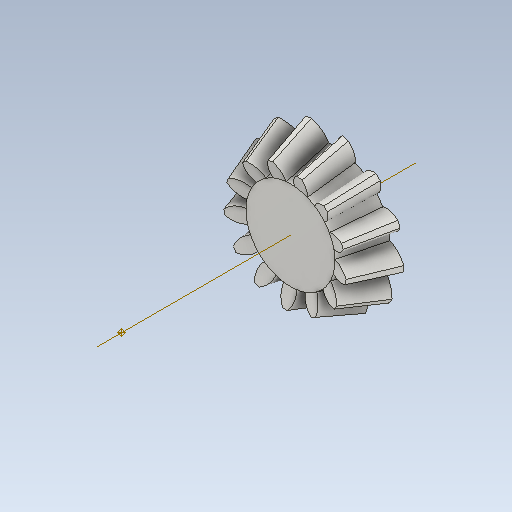
# Autodesk Inventor part: Kegelrad1
Saved by Autodesk Inventor 2021 (Build 250183000, 183)
## iProperties
CustomPartVersion: 1
Created: 2021-01-28
Part Number: Kegelrad1
Material: Steel, Mild
Document SubType Name: Modeling
Designer: LETPJG
Categories: <?xml version="1.0" encoding="UTF-16"?> <MemberInstance><Categories><FamilyTemplate><FamilyTemplateParameter ValueType="xs:double" Id="1" ObjectReferenceKey="da_z" ObjectType="kUserParameterObject"/><FamilyTemplateParameter ValueType="xs:double" Id="2" ObjectReferenceKey="da_b" ObjectType="kUserParameterObject"/><FamilyTemplateParameter ValueType="xs:double" Id="3" ObjectReferenceKey="da_beta" ObjectType="kUserParameterObject"/><FamilyTemplateParameter ValueType="xs:double" Id="4" ObjectReferenceKey="da_dae" ObjectType="kUserParameterObject"/><FamilyTemplateParameter ValueType="xs:double" Id="5" ObjectReferenceKey="da_ve" ObjectType="kUserParameterObject"/><FamilyTemplateParameter ValueType="xs:double" Id="6" ObjectReferenceKey="da_omega" ObjectType="kUserParameterObject"/><FamilyTemplateParameter ValueType="xs:string" Id="7" ObjectReferenceKey="EAIAABAAAAAAHwAAAAAAAIAAAAAAAAAA" ObjectType="83914240" SubObjectId="SurfaceGeometry"/></FamilyTemplate><ParamToTemplateMap><ParamToTemplate CategoryParameter="//CategoryParameter[@InternalName='046C89C9-8512-4d59-83FE-43B91F4F132A']" TemplateParameter="1"/><ParamToTemplate CategoryParameter="//CategoryParameter[@InternalName='2552DF32-E462-4b46-AEBF-C6C7768E72AC']" TemplateParameter="2"/><ParamToTemplate CategoryParameter="//CategoryParameter[@InternalName='C9EE641D-15FC-4fae-A226-E94C4372FDD7']" TemplateParameter="3"/><ParamToTemplate><ParamToTemplate CategoryParameter="//CategoryParameter[@InternalName='00B6519A-459B-49c7-AD84-2E56D39A5744']" ConstantValue="0.000000"/></ParamToTemplate><ParamToTemplate><ParamToTemplate CategoryParameter="//CategoryParameter[@InternalName='04B31F0E-C7A6-4894-AA32-9629BEFACF47']" ConstantValue="1.000000"/></ParamToTemplate><ParamToTemplate><ParamToTemplate CategoryParameter="//CategoryParameter[@InternalName='43CBEC2E-7847-49e7-A936-2F7889FCB2D9']" ConstantValue="0.200000"/></ParamToTemplate><ParamToTemplate><ParamToTemplate CategoryParameter="//CategoryParameter[@InternalName='B1EFC894-105D-4ebd-86BF-FA20ED196853']" ConstantValue="0.300000"/></ParamToTemplate><ParamToTemplate><ParamToTemplate CategoryParameter="//CategoryParameter[@InternalName='51175063-3D10-4879-93E8-6246FE8B403D']" ConstantValue="2060000000.000000"/></ParamToTemplate><ParamToTemplate><ParamToTemplate CategoryParameter="//CategoryParameter[@InternalName='A3A52E27-4454-46a9-B0BD-C932399B70AF']" ConstantValue="0.300000"/></ParamToTemplate><ParamToTemplate CategoryParameter="//CategoryParameter[@InternalName='2A200944-5A8C-41ca-B96E-8520D2E510F1']" TemplateParameter="4"/><ParamToTemplate><ParamToTemplate CategoryParameter="//CategoryParameter[@InternalName='1A637F62-92C8-44bc-B81F-10802510B579']" ConstantValue="1.175421"/></ParamToTemplate><ParamToTemplate CategoryParameter="//CategoryParameter[@InternalName='B52DD4BE-6863-48fb-BF58-89EF6F9EC65C']" TemplateParameter="5"/><ParamToTemplate><ParamToTemplate CategoryParameter="//CategoryParameter[@InternalName='3956BFF2-84D2-457d-93C2-9B0613DEBA67']" ConstantValue="1.568105"/></ParamToTemplate><ParamToTemplate CategoryParameter="//CategoryParameter[@InternalName='739CFA02-461B-4bf8-8049-181FCAD8B28F']" TemplateParameter="6"/><ParamToTemplate><ParamToTemplate CategoryParameter="//CategoryParameter[@InternalName='A27E999F-E2CE-4481-8A2A-EBF499C4C3C5']" ConstantValue="0.000000"/></ParamToTemplate><ParamToTemplate><ParamToTemplate CategoryParameter="//CategoryParameter[@InternalName='9E1B4470-B2D3-4ff1-B813-535BB4CDF51A']" ConstantValue="3520000.000000"/></ParamToTemplate><ParamToTemplate><ParamToTemplate CategoryParameter="//CategoryParameter[@InternalName='F8452263-BFF6-458c-9FB1-07C4B99E95CD']" ConstantValue="11400000.000000"/></ParamToTemplate><ParamToTemplate><ParamToTemplate CategoryParameter="//CategoryParameter[@InternalName='3E3BB259-FD49-497f-8171-6EBC954A3479']" ConstantValue="2.000000"/></ParamToTemplate><ParamToTemplate CategoryParameter="//CategoryParameter[@InternalName='27C3BAF2-7550-4e4b-AE2C-0DB134B7D9B7']" TemplateParameter="7"/></ParamToTemplateMap><Category DisplayName="Gear" InternalName="DC85795E-93AB-48d5-8EEE-5A27447B64BD" Mnemonic="Gear"><CategoryParameter DisplayName="z" InternalName="046C89C9-8512-4d59-83FE-43B91F4F132A" Mnemonic="z"/><CategoryParameter DisplayName="b" InternalName="2552DF32-E462-4b46-AEBF-C6C7768E72AC" Mnemonic="b"/><CategoryParameter DisplayName="||b|" InternalName="C9EE641D-15FC-4fae-A226-E94C4372FDD7" Mnemonic="beta"/><CategoryParameter DisplayName="x" InternalName="00B6519A-459B-49c7-AD84-2E56D39A5744" Mnemonic="x"/><CategoryParameter DisplayName="a*" InternalName="04B31F0E-C7A6-4894-AA32-9629BEFACF47" Mnemonic="a"/><CategoryParameter DisplayName="c*" InternalName="43CBEC2E-7847-49e7-A936-2F7889FCB2D9" Mnemonic="c"/><CategoryParameter DisplayName="r|.f|*" InternalName="B1EFC894-105D-4ebd-86BF-FA20ED196853" Mnemonic="rf"/><CategoryParameter DisplayName="E" InternalName="51175063-3D10-4879-93E8-6246FE8B403D" Mnemonic="E"/><CategoryParameter DisplayName="||m|" InternalName="A3A52E27-4454-46a9-B0BD-C932399B70AF" Mnemonic="mi"/><Category DisplayName="BevelGear" InternalName="0C98F69A-0C2B-4791-B2FE-7691BB227E77" Mnemonic="BevelGear"><CategoryParameter DisplayName="d|.ae|" InternalName="2A200944-5A8C-41ca-B96E-8520D2E510F1" Mnemonic="dae"/><CategoryParameter DisplayName="d|.ai|" InternalName="1A637F62-92C8-44bc-B81F-10802510B579" Mnemonic="dai"/><CategoryParameter DisplayName="A|.e|" InternalName="B52DD4BE-6863-48fb-BF58-89EF6F9EC65C" Mnemonic="ve"/><CategoryParameter DisplayName="A|.i|" InternalName="3956BFF2-84D2-457d-93C2-9B0613DEBA67" Mnemonic="vi"/><CategoryParameter DisplayName="||S|" InternalName="739CFA02-461B-4bf8-8049-181FCAD8B28F" Mnemonic="omega"/><CategoryParameter DisplayName="x|.t|" InternalName="A27E999F-E2CE-4481-8A2A-EBF499C4C3C5" Mnemonic="xt"/><CategoryParameter DisplayName="||s||.Flim|" InternalName="9E1B4470-B2D3-4ff1-B813-535BB4CDF51A" Mnemonic="sFlim"/><CategoryParameter DisplayName="||s||.Hlim|" InternalName="F8452263-BFF6-458c-9FB1-07C4B99E95CD" Mnemonic="sHlim"/><CategoryParameter DisplayName="Typ" InternalName="3E3BB259-FD49-497f-8171-6EBC954A3479" Mnemonic="type"/><CategoryParameter DisplayName="PitchDiameter" InternalName="27C3BAF2-7550-4e4b-AE2C-0DB134B7D9B7" Mnemonic="IDS_PITCHDIAM"/></Category></Category></Categories></MemberInstance>
Mass: 60.9118 g
Surface Area: 34.3074 cm^2
Volume: 7.7496 cm^3
Density: 7.86 g/cm^3
Appearance: Steel
d48: 0,000 mm
d49: 0,000 mm
d50: 90,00 grd
d52: 0,000 mm
d53: 0,000 mm
d54: 0,00 grd
Author: LETPJG
Autodesk Inventor part; units mm, degrees
ref_plane "Netzebene2" through (0, 0, 0) normal (0.9709418, 0.2393157, 0) x (0, 0, 1)
sketch "Skizze des Zahnradkörpers" plane through (0, 0, 0) normal (1, 0, 0) x (0, 1, 0)
  line L0 (0, 0) -> (5.358759, -20.370903) construction
  line L1 (5.358759, -20.370903) -> (7.387682, -19.711503)
  line L2 (7.387682, -19.711503) -> (0, 0) construction
  line L3 (6.5, -20) -> (0, 0) construction
  line L4 (4.263041, -16.205617) -> (5.877106, -15.681046)
  line L5 (5.358759, -20.370903) -> (4.263041, -16.205617)
  line L6 (7.387682, -19.711503) -> (5.877106, -15.681046)
  line L7 (0, -39.386751) -> (0, 6.564458)
  line L8 (0, -20) -> (7.387682, -20) construction
  dimension "d0" = 13
  dimension "d1" = 10.71752
  dimension "d2" = 14.77536
  dimension "d3" = 4.3
  dimension "d4" = 19.7115
  constraints: 16 end point, 4 point on line, 3 perpendicular, 2 collinear, 1 horizontal alignment, 1 vertical alignment
  measures "d0" diameter of L3.start L7
  measures "d1" diameter of L0.end L7
  measures "d2" diameter of L1.end L7
  measures "d3" distance between parallel lines of L1 L4
  measures "d4" vertical distance of L1.end L0.start
revolve "Zahnradkörper" add sketch "Skizze des Zahnradkörpers" angle 360 about axis through (0, 0, 0) along (0, 0, 1)
ref_plane "Zahnebene" through (0, 6.5, -20) normal (0, -0.3090861, 0.9510341) x (1, 0, 0)
sketch "Startskizze" plane through (0, 6.5, -20) normal (0, -0.3090861, 0.9510341) x (1, 0, 0)
  line L0 (0, -23.505131) -> (0, 10.644758)
  arc A0 (-0.515171, -1.456006) -> (-2.356776, 1.236345) centre (-3.066949, -1.22544) ccw
  arc A1 (2.356776, 1.236345) -> (0.515171, -1.456006) centre (3.066949, -1.22544) ccw
  line L1 (-0.515171, -1.456006) -> (0.515171, -1.456006)
  arc A2 (2.356776, 1.236345) -> (-2.356776, 1.236345) centre (0, -6.834666) ccw
  dimension "d7" = 2.56217
  dimension "d8" = 3.06695
  dimension "d9" = 5.60923
  dimension "d57" = 8.40807
  dimension "d58" = 5.37866
  constraints: 6 point on circle, 3 centre point, 3 symmetric about line, 2 end point, 1 coincident, 1 perpendicular, 1 other
  measures "d7" radius of A0
  measures "d8" horizontal distance of point (0, -6.835) A0.centre
  measures "d9" vertical distance of point (0, -6.835) A0.centre
  measures "d57" radius of A2
  measures "d58" distance from line of A2.centre L1
ref_plane "Endebene" through (0, 5.13796, -15.809107) normal (0, -0.3090861, 0.9510341) x (1, 0, 0)
sketch "Endskizze" plane through (0, 5.13796, -15.809107) normal (0, -0.3090861, 0.9510341) x (1, 0, 0)
  line L0 (0, -15.35404) -> (0, 6.953444)
  arc A0 (-0.40722, -1.150908) -> (-1.862926, 0.977276) centre (-2.424286, -0.968655) ccw
  arc A1 (1.862926, 0.977276) -> (0.40722, -1.150908) centre (2.424286, -0.968655) ccw
  line L1 (-0.40722, -1.150908) -> (0.40722, -1.150908)
  arc A2 (1.862926, 0.977276) -> (-1.862926, 0.977276) centre (0, -5.402498) ccw
  dimension "d12" = 2.02528
  dimension "d15" = 2.42429
  dimension "d16" = 4.43384
  dimension "d59" = 6.6462
  dimension "d60" = 4.25159
  constraints: 6 point on circle, 3 centre point, 3 symmetric about line, 2 end point, 1 coincident, 1 other
  measures "d12" radius of A0
  measures "d15" horizontal distance of A0.centre point (0, -5.402)
  measures "d16" vertical distance of A0.centre point (0, -5.402)
  measures "d59" radius of A2
  measures "d60" distance from line of A2.centre L1
loft "Loft" cut profiles "Startskizze", "Endskizze"
pattern_circular "Circular Pattern" count 13 over 360 about axis through (0, 0, 0) along (0, 0, 1) of "Loft"
sketch3d "3D-Skizze rechts"
ref_plane "Endebene rechts" through (-1.394472, 4.945107, -15.809107) normal (0.0838877, -0.2974845, 0.9510341) x (0.962465, 0.2714057, 0)
sketch "Endskizze rechts" plane through (-1.394472, 4.945107, -15.809107) normal (0.0838877, -0.2974845, 0.9510341) x (0.962465, 0.2714057, 0)
  arc A0 (-0.40722, -1.150908) -> (-1.862926, 0.977276) centre (-2.424286, -0.968655) ccw
  line L0 (0, -19.937006) -> (0, 11.536399)
  arc A1 (1.862926, 0.977276) -> (0.40722, -1.150908) centre (2.424286, -0.968655) ccw
  line L1 (-0.40722, -1.150908) -> (0.40722, -1.150908)
  arc A2 (1.862926, 0.977276) -> (-1.862926, 0.977276) centre (0, -5.402498) ccw
  dimension "d70" = 2.42429
  dimension "d71" = 4.43384
  dimension "d72" = 2.02528
  dimension "d73" = 4.25159
  dimension "d74" = 6.6462
  constraints: 6 point on circle, 3 centre point, 3 symmetric about line, 2 end point, 1 coincident, 1 perpendicular, 1 other
  measures "d70" horizontal distance of A2.centre A0.centre
  measures "d71" vertical distance of point (0, -5.402) A0.centre
  measures "d72" radius of A0
  measures "d73" distance from line of point (0, -5.402) L1
  measures "d74" radius of A2
feature "Erhebung rechts" [suppressed]
pattern_circular "Runde Anordnung rechts" [suppressed]
sketch3d "3D-Skizze links"
ref_plane "Endebene links" through (1.399335, 4.945107, -15.810729) normal (-0.0841704, -0.2974496, 0.95102) x (0.9622174, -0.2722822, 0)
sketch "Endskizze links" plane through (1.399335, 4.945107, -15.810729) normal (-0.0841704, -0.2974496, 0.95102) x (0.9622174, -0.2722822, 0)
  line L0 (0, -34.877335) -> (0, 17.854612)
  arc A0 (-0.40722, -1.151664) -> (-1.862926, 0.97652) centre (-2.424286, -0.969412) ccw
  arc A1 (1.862926, 0.97652) -> (0.40722, -1.151664) centre (2.424286, -0.969412) ccw
  line L1 (-0.40722, -1.151664) -> (0.40722, -1.151664)
  ellipse E0 centre (0, -4.847471) end of major axis (5.877106, -4.847471) minor radius 5.589245
  arc A2 (1.862926, 0.97652) -> (-1.862926, 0.97652) centre (0, -5.403254) ccw
  dimension "d56" = 5.58925
  dimension "d30" = 2.02528
  dimension "d31" = 2.42429
  dimension "d32" = 4.43384
  dimension "d61" = 6.6462
  dimension "d62" = 4.25159
  constraints: 6 point on circle, 3 centre point, 3 symmetric about line, 2 end point, 1 coincident, 2 other
  measures "d30" radius of A0
  measures "d31" horizontal distance of point (0, -5.403) A0.centre
  measures "d32" vertical distance of A0.centre point (0, -5.403)
  measures "d61" radius of A2
  measures "d62" distance from line of point (0, -5.403) L1
feature "Erhebung links" [suppressed]
pattern_circular "Runde Anordnung links" [suppressed]
sketch "Körperskizze" plane through (0, 0, 0) normal (1, 0, 0) x (0, 1, 0)
  line L0 (0, -35.037536) -> (0, -19.530831)
  line L1 (5.358759, -20.370903) -> (4.263041, -16.205617)
  line L2 (4.263041, -16.205617) -> (0, -16.205617)
  line L3 (5.358759, -20.370903) -> (0, -20.370903)
  constraints: 4 end point, 2 perpendicular, 2 point on line
sketch "Körperskizze outline for Festkörper" plane through (0, 0, 0) normal (1, 0, 0) x (0, 1, 0)
  line L0 (0, -20.370903) -> (5.358759, -20.370903)
  line L1 (0, -16.205617) -> (0, -20.370903)
  line L2 (4.263041, -16.205617) -> (0, -16.205617)
  line L3 (5.358759, -20.370903) -> (4.263041, -16.205617)
revolve "Festkörper" add sketch "Körperskizze outline for Festkörper" angle 360 about axis through (0, 0, 0) along (0, 0, 1)
sketch "Sketch6" plane through (0, 0, 0) normal (1, 0, 0) x (0, 1, 0)
  line L0 (6.5, -20) -> (0, 0)
  line L1 (0, -37.799919) -> (0, 6.299986)
surface revolve "Flankendurchmesser" sketch "Sketch6" angle 360 about axis through (0, 0, 0) along (0, 0, 1) shown no curves L0
equation "\"d0\" = da_de"
equation "\"d1\" = da_dfe"
equation "\"d2\" = da_dae"
equation "\"d3\" = da_b"
equation "\"d4\" = da_ve"
equation "\"d7\" = fd_rr"
equation "\"d8\" = fd_x"
equation "\"d9\" = fd_y"
equation "\"d57\" = 0.5 * fd_dva + 0.3 * da_he"
equation "\"d58\" = 0.5 * fd_dva - 1.12 * da_he"
equation "\"da_teethtype\" = 0"
equation "\"da_b\" = 4.3"
equation "\"da_de\" = 13"
equation "\"da_dae\" = 14.77536"
equation "\"da_dfe\" = 10.71752"
equation "\"da_le\" = 21.02974"
equation "\"da_omega\" = 90deg"
equation "\"da_beta\" = 0"
equation "\"da_delta\" = 18.004162deg"
equation "\"da_alpha\" = 20deg"
equation "\"da_he\" = 2.13339"
equation "\"da_ve\" = 19.7115"
equation "\"da_zv\" = 13.669332"
equation "\"fd_loft\" = da_b + 0.05 * da_he"
equation "\"fd_x\" = fd_x1 + fd_x2"
equation "\"fd_y\" = fd_y1 - fd_y2"
equation "\"fd_dd\" = fd_dva - 0.8 * da_he"
equation "\"da_dvw\" = 13.66933"
equation "\"d11\" = fd_loft"
equation "\"da_dm\" = 11.67093"
equation "\"da_x\" = 0"
equation "\"da_m\" = 1"
equation "\"d50\" = da_omega"
equation "\"fd_rr\" = 2.562173"
equation "\"fd_dva\" = 15.536105"
equation "\"fd_x1\" = 0.792339"
equation "\"fd_x2\" = 2.27461"
equation "\"fd_y1\" = 6.788583"
equation "\"fd_y2\" = 1.179357"
body "Solid1"
body "Srf1"
